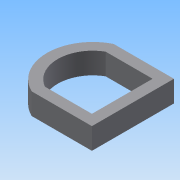
# Autodesk Inventor part: truck_sizings
Saved by Autodesk Inventor 2015 (Build 190159000, 159)
## iProperties
Created: 2016-01-21
Part Number: truck_sizings
Material: Generic
Document SubType Name: Modeling
Designer: JoshuaYuan
Density: 1 g/cm^3
Appearance: Default
Author: JoshuaYuan
Autodesk Inventor part; units mm, degrees
ref_plane "YZ Plane" through (0, 0, 0) normal (1, 0, 0) x (0, 1, 0)
ref_plane "XZ Plane" through (0, 0, 0) normal (0, 1, 0) x (-1, 0, 0)
ref_plane "XY Plane" through (0, 0, 0) normal (0, 0, 1) x (1, 0, 0)
sketch "Sketch1" plane through (0, 0, 0) normal (0, 1, 0) x (-1, 0, 0)
  line L0 (53.0453, 125.5248) -> (39.0753, 125.5248)
  line L1 (39.0753, 125.5248) -> (39.0753, 107.4908)
  line L2 (39.0753, 107.4908) -> (53.0453, 107.4908)
  arc A0 (53.0453, 107.4908) -> (53.0453, 125.5248) centre (47.8352, 116.5078) ccw
  line L3 (51.0559, 55.1199) -> (37.0859, 55.1199)
  line L4 (37.0859, 55.1199) -> (37.0859, 37.0859)
  line L5 (37.0859, 37.0859) -> (51.0559, 37.0859)
  arc A1 (51.0559, 37.0859) -> (51.0559, 55.1199) centre (39.6314, 46.1029) ccw
  line L6 (61.7452, 17.3999) -> (47.7752, 17.3999)
  line L7 (47.7752, 17.3999) -> (47.7752, -0.6341)
  line L8 (47.7752, -0.6341) -> (61.7452, -0.6341)
  arc A2 (61.7452, -0.6341) -> (61.7452, 17.3999) centre (49.459, 8.3829) ccw
  line L9 (89.1373, 73.7746) -> (75.1673, 73.7746)
  line L10 (75.1673, 73.7746) -> (75.1673, 55.7406)
  line L11 (75.1673, 55.7406) -> (89.1373, 55.7406)
  arc A3 (89.1373, 55.7406) -> (89.1373, 73.7746) centre (83.9272, 64.7576) ccw
  line L12 (52.5031, 58.2949) -> (33.9109, 58.2949)
  line L13 (33.9109, 58.2949) -> (33.9109, 33.9109)
  line L14 (33.9109, 33.9109) -> (52.5031, 33.9109)
  arc A4 (52.5031, 33.9109) -> (52.5031, 58.2949) centre (39.6314, 46.1029) ccw
  line L15 (53.8365, 128.6998) -> (35.9003, 128.6998)
  line L16 (35.9003, 128.6998) -> (35.9003, 104.3158)
  line L17 (35.9003, 104.3158) -> (53.8365, 104.3158)
  arc A5 (53.8365, 104.3158) -> (53.8365, 128.6998) centre (47.8352, 116.5078) ccw
  line L18 (63.26, 20.5749) -> (44.6002, 20.5749)
  line L19 (44.6002, 20.5749) -> (44.6002, -3.8091)
  line L20 (44.6002, -3.8091) -> (63.26, -3.8091)
  arc A6 (63.26, -3.8091) -> (63.26, 20.5749) centre (49.459, 8.3829) ccw
  line L21 (89.9285, 52.5656) -> (71.9923, 52.5656)
  line L22 (71.9923, 52.5656) -> (71.9923, 76.9496)
  line L23 (71.9923, 76.9496) -> (89.9285, 76.9496)
  arc A7 (89.9285, 52.5656) -> (89.9285, 76.9496) centre (83.9272, 64.7576) ccw
  point P0 (0, 0)
  dimension "d0" = 10.414
  dimension "d1" = 13.97
  dimension "d2" = 18.034
  dimension "d3" = 14.5542
  dimension "d4" = 13.97
  dimension "d5" = 18.034
  dimension "d6" = 15.24
  dimension "d7" = 13.97
  dimension "d8" = 18.034
  dimension "d10" = 13.97
  dimension "d11" = 18.034
  dimension "d13" = 3.175
  dimension "d14" = 3.175
  dimension "d15" = 3.175
  dimension "d19" = 10.414
  dimension "d20" = 3.175
  constraints: 48 end point, 16 perpendicular, 16 point on circle, 8 centre point, 4 horizontal, 4 parallel, 12 other
  measures "d0" radius of A0
  measures "d1" distance of L1.end L2.end
  measures "d2" distance of L0.end L1.end
  measures "d3" radius of A1
  measures "d4" distance of L4.end L5.end
  measures "d5" distance of L3.end L4.end
  measures "d6" radius of A2
  measures "d7" distance of L7.end L8.end
  measures "d8" distance of L6.end L7.end
  measures "d10" distance of L10.end L11.end
  measures "d11" distance of L9.end L10.end
  measures "d13" distance between parallel lines of L15 L0
  measures "d14" distance between parallel lines of L12 L3
  measures "d15" distance between parallel lines of L18 L6
  measures "d19" radius of A3
  measures "d20" distance between parallel lines of L11 L21
extrude "Extrusion2" add sketch "Sketch1" along normal blind 6.35 contours A5 L17 L16 L15
body "Solid2"
